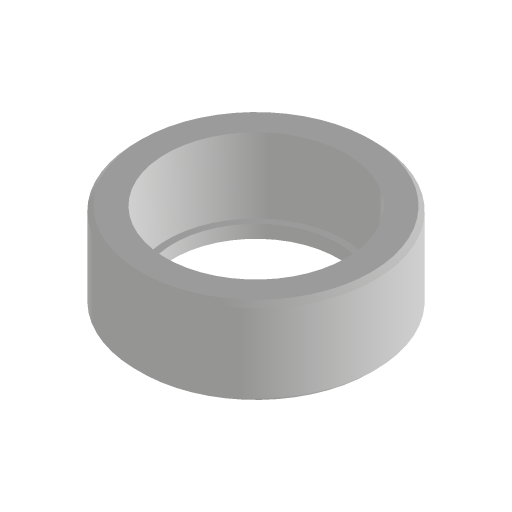
# Autodesk Inventor part: NAUO43_Tubelens_156.5_Astromedia
Saved by Autodesk Inventor 2024.1 (Build 281209000, 209)
## iProperties
Created: 2024-05-28
Part Number: NAUO43_Tubelens_156.5_Astromedia
Material: Generisch
Document SubType Name: Modeling
Designer: diederichbenedict
Density: 1 g/cm^3
Appearance: Vorgabe
Author: diederichbenedict
Autodesk Inventor part; units mm, degrees
ref_plane "YZ Plane" through (0, 0, 0) normal (1, 0, 0) x (0, 1, 0)
ref_plane "XZ Plane" through (0, 0, 0) normal (0, 1, 0) x (-1, 0, 0)
ref_plane "XY Plane" through (0, 0, 0) normal (0, 0, 1) x (1, 0, 0)
sketch "Skizze1" plane through (0, 0, 0) normal (0, 1, 0) x (-1, 0, 0)
  line L0 (-20.4476, 0) -> (-20.7967, 20)
  line L1 (-20.4476, 0) -> (-0.4446, 0) construction
  line L2 (-20.7967, 20) -> (-27.5, 20)
  line L3 (-27.5, 20) -> (-27.5, 0)
  line L4 (0, -4) -> (0, 24) projected
  line L5 (-20.4476, 0) -> (-27.5, 0)
  line L6 (5.5, 0) -> (-33, 0) projected
  line L7 (0, -4) -> (0, 24) projected
  line L8 (-20.5, 0) -> (-19, 0)
  line L9 (-19, 0) -> (-19, 3)
  line L10 (-19, 3) -> (-20.5, 3)
  line L11 (-20.5, 3) -> (-20.5, 0)
  point P0 (0, 0)
  dimension "d1" = 91
  dimension "d2" = 0
  dimension "d4" = 0
  dimension "d6" = 20
  dimension "d9" = 27.5
  dimension "d10" = 3
  dimension "d11" = 19
  dimension "d12" = 20.5
  constraints: 18 end point, 3 horizontal, 2 parallel, 2 perpendicular, 2 point on line, 1 collinear, 1 equal length
  measures "d1" angle of L1 L0
  measures "d2" angle of L3 L4
  measures "d4" distance from line of point (0, 0) L5
  measures "d6" distance of L3.end L2.end
  measures "d9" distance from line of L3 point (0, 0)
  measures "d10" distance of L9.end L8.end
  measures "d11" distance of L8.end point (0, 0)
  measures "d12" horizontal distance of point (0, 0) L10.end
revolve "Umdrehung1" add sketch "Skizze1" angle 360 about axis through (0, 0, -10) along (0, 0, 1)
chamfer "Fasen1" distance 1 angle 45 2 edges at (-27.5, 0, 20) (-27.5, 0, 0)
